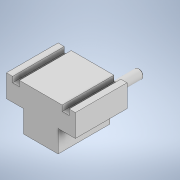
# Autodesk Inventor part: Z_axis
Saved by Autodesk Inventor 2020 (Build 240168000, 168)
## iProperties
Created: 2020-05-03
Part Number: Z_axis
Material: Generic
Document SubType Name: Modeling
Designer: zhang
Density: 1 g/cm^3
Appearance: Default
Author: zhang
Autodesk Inventor part; units mm, degrees
ref_plane "YZ Plane" through (0, 0, 0) normal (1, 0, 0) x (0, 1, 0)
ref_plane "XZ Plane" through (0, 0, 0) normal (0, 1, 0) x (-1, 0, 0)
ref_plane "Work Plane1" through (0, 0, 200) normal (0, 0, 1) x (1, 0, 0)
sketch "Sketch1" plane through (0, 0, 200) normal (0, 0, 1) x (1, 0, 0)
  line L0 (0, 8.259) -> (0, -5.5938)
  line L1 (-6.2911, 0) -> (6.8799, 0)
  line L2 (0, 94) -> (-100, 94)
  line L3 (-100, 94) -> (-100, 29)
  line L4 (-100, 29) -> (-50, 29)
  line L5 (-50, 29) -> (-50, -35)
  line L6 (-50, -35) -> (0, -35)
  line L7 (0, 94) -> (100, 94)
  line L8 (100, 94) -> (100, 29)
  line L9 (100, 29) -> (50, 29)
  line L10 (50, 29) -> (50, -35)
  line L11 (50, -35) -> (0, -35)
  point P0 (0, 0)
  dimension "d1" = 100
  dimension "d2" = 188
  dimension "d3" = 65
  dimension "d5" = 50
  dimension "d21" = 64
  constraints: 24 end point, 4 perpendicular, 4 symmetric about line, 3 horizontal, 2 point on line, 2 vertical
  measures "d1" distance of L2.start L2.end
  measures "d2" diameter of L2 L1
  measures "d3" distance between parallel lines of L4 L2
  measures "d5" distance of L3.end L4.end
  measures "d21" distance of L4.end L5.end
extrude "Extrusion1" add sketch "Sketch1" along normal blind 150
sketch "Sketch2" plane through (0, 0, 200) normal (0, 0, 1) x (1, 0, 0)
  circle A0 centre (0, 0) radius 13
  dimension "d8" = 26
  constraints: 1 centre point, 1 coincident
  measures "d8" diameter of A0
extrude "Extrusion2" add sketch "Sketch2" against normal blind 135
sketch "Sketch3" plane through (0, 0, 200) normal (0, 0, -1) x (-1, 0, 0)
  line L0 (20, -20) -> (-20, -20)
  line L1 (-20, -20) -> (-20, 20)
  line L2 (-20, 20) -> (20, 20)
  line L3 (20, 20) -> (20, -20)
  line L4 (0, -60.8) -> (0, 119.8) projected
  line L5 (140, 0) -> (-140, 0) projected
  point P0 (0, 0)
  dimension "d11" = 40
  dimension "d12" = 40
  constraints: 8 end point, 2 parallel, 1 horizontal, 1 perpendicular, 2 other
  measures "d11" distance of L0.end L1.end
  measures "d12" distance of L0.start L0.end
extrude "Extrusion3" add sketch "Sketch3" along normal blind 60
chamfer "Chamfer1" distance 5 angle 45 4 edges at (-20, -20, 170) (-20, 20, 170) (20, -20, 170) (20, 20, 170)
chamfer "Chamfer2" distance 2 angle 45 1 edges at (-13, 0, 65)
sketch "Sketch4" plane through (0, 0, 350) normal (0, 0, 1) x (1, 0, 0)
  line L0 (0, -53.3893) -> (0, 113.7531)
  line L1 (100, 94) -> (-100, 94) projected
  line L2 (82, 94) -> (62, 94)
  line L3 (62, 94) -> (62, 78)
  line L4 (62, 78) -> (82, 78)
  line L5 (82, 78) -> (82, 94)
  line L6 (100, 29) -> (100, 94) projected
  line L7 (-82, 94) -> (-62, 94)
  line L8 (-62, 94) -> (-62, 78)
  line L9 (-62, 78) -> (-82, 78)
  line L10 (-82, 78) -> (-82, 94)
  point P0 (0, 0)
  dimension "d22" = 20
  dimension "d23" = 16
  dimension "d24" = 18
  constraints: 18 end point, 4 symmetric about line, 2 parallel, 2 vertical, 1 horizontal, 1 perpendicular, 1 point on line
  measures "d22" distance of L3.end L4.end
  measures "d23" distance of L2.end L3.end
  measures "d24" distance between parallel lines of L6 L5
extrude "Extrusion4" cut sketch "Sketch4" against normal through all
body "Solid1"
